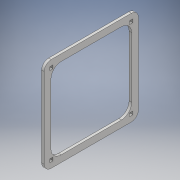
# Autodesk Inventor part: FrontPanelSquishything
Saved by Autodesk Inventor 2017 (Build 210142000, 142)
## iProperties
Created: 2019-07-06
Part Number: FrontPanelSquishything
Material: Generic
Document SubType Name: Modeling
Designer: DDeGo
Density: 1 g/cm^3
Appearance: Default
Author: DDeGo
Autodesk Inventor part; units mm, degrees
ref_plane "YZ Plane" through (0, 0, 0) normal (1, 0, 0) x (0, 1, 0)
ref_plane "XZ Plane" through (0, 0, 0) normal (0, 1, 0) x (-1, 0, 0)
ref_plane "XY Plane" through (0, 0, 0) normal (0, 0, 1) x (1, 0, 0)
sketch "Sketch1" plane through (0, 0, 0) normal (1, 0, 0) x (0, 1, 0)
  line L0 (0, 13.5) -> (156.2, 13.5)
  line L1 (169.7, 0) -> (169.7, -156.2)
  line L2 (156.2, -169.7) -> (0, -169.7)
  line L3 (-13.5, -156.2) -> (-13.5, 0)
  arc A0 (169.7, 0) -> (156.2, 13.5) centre (156.2, 0) ccw
  arc A1 (156.2, -169.7) -> (169.7, -156.2) centre (156.2, -156.2) ccw
  arc A2 (-13.5, -156.2) -> (0, -169.7) centre (0, -156.2) ccw
  arc A3 (0, 13.5) -> (-13.5, 0) centre (0, 0) ccw
  line L4 (19.5, 0.5) -> (136.7, 0.5)
  line L5 (156.7, -19.5) -> (156.7, -136.7)
  line L6 (136.7, -156.7) -> (19.5, -156.7)
  line L7 (-0.5, -136.7) -> (-0.5, -19.5)
  arc A4 (19.5, 0.5) -> (-0.5, -19.5) centre (19.5, -19.5) ccw
  arc A5 (-0.5, -136.7) -> (19.5, -156.7) centre (19.5, -136.7) ccw
  arc A6 (136.7, -156.7) -> (156.7, -136.7) centre (136.7, -136.7) ccw
  arc A7 (156.7, -19.5) -> (136.7, 0.5) centre (136.7, -19.5) ccw
  dimension "d0" = 13.5
  dimension "d1" = 183.2
  dimension "d2" = 183.2
  dimension "d15" = 13
  dimension "d16" = 13
  dimension "d17" = 13
  dimension "d18" = 13
  dimension "d19" = 20
  constraints: 16 end point, 16 point on circle, 16 tangent, 8 centre point, 6 equal radius, 4 parallel, 2 horizontal, 2 perpendicular, 1 other
  measures "d0" radius of A0
  measures "d1" distance between parallel lines of L2 L0
  measures "d2" distance between parallel lines of L1 L3
  measures "d15" distance between parallel lines of L3 L7
  measures "d16" distance between parallel lines of L0 L4
  measures "d17" distance between parallel lines of L1 L5
  measures "d18" distance between parallel lines of L2 L6
  measures "d19" radius of A4
extrude "Extrusion1" add sketch "Sketch1" along normal blind 5
sketch "Sketch2" plane through (0, 0, 0) normal (-1, 0, 0) x (0, 0, 1)
  line L0 (-0.5, 155.7) -> (-155.7, 155.7) construction
  line L1 (-155.7, 155.7) -> (-155.7, 0.5) construction
  line L2 (-155.7, 0.5) -> (-0.5, 0.5) construction
  line L3 (-0.5, 0.5) -> (-0.5, 155.7) construction
  line L4 (2.625, 152.575) -> (-3.625, 152.575)
  line L5 (-3.625, 152.575) -> (-3.625, 158.825)
  line L6 (-3.625, 158.825) -> (2.625, 158.825)
  line L7 (2.625, 158.825) -> (2.625, 152.575)
  line L8 (2.625, 152.575) -> (-3.625, 158.825) construction
  line L9 (-3.625, 152.575) -> (2.625, 158.825) construction
  line L10 (-3.625, 3.625) -> (2.625, 3.625)
  line L11 (2.625, 3.625) -> (2.625, -2.625)
  line L12 (2.625, -2.625) -> (-3.625, -2.625)
  line L13 (-3.625, -2.625) -> (-3.625, 3.625)
  line L14 (-3.625, 3.625) -> (2.625, -2.625) construction
  line L15 (2.625, 3.625) -> (-3.625, -2.625) construction
  line L16 (-158.825, 3.625) -> (-152.575, 3.625)
  line L17 (-152.575, 3.625) -> (-152.575, -2.625)
  line L18 (-152.575, -2.625) -> (-158.825, -2.625)
  line L19 (-158.825, -2.625) -> (-158.825, 3.625)
  line L20 (-158.825, 3.625) -> (-152.575, -2.625) construction
  line L21 (-152.575, 3.625) -> (-158.825, -2.625) construction
  line L22 (-152.575, 152.575) -> (-158.825, 152.575)
  line L23 (-158.825, 152.575) -> (-158.825, 158.825)
  line L24 (-158.825, 158.825) -> (-152.575, 158.825)
  line L25 (-152.575, 158.825) -> (-152.575, 152.575)
  line L26 (-152.575, 152.575) -> (-158.825, 158.825) construction
  line L27 (-158.825, 152.575) -> (-152.575, 158.825) construction
  line L28 (-156.2, -13.5) -> (0, -13.5) projected
  line L29 (13.5, 0) -> (13.5, 156.2) projected
  line L30 (0, 169.7) -> (-156.2, 169.7) projected
  line L31 (-169.7, 156.2) -> (-169.7, 0) projected
  point P0 (0, 0)
  dimension "d20" = 6.25
  dimension "d21" = 6.25
  dimension "d22" = 14
  dimension "d23" = 14
  dimension "d24" = 14
  dimension "d25" = 14
  constraints: 56 end point, 10 parallel, 8 midpoint, 6 equal length, 5 horizontal, 5 perpendicular
  measures "d20" distance of L5.end L6.end
  measures "d21" distance of L6.end L4.start
  measures "d22" distance between parallel lines of L28 L2
  measures "d23" distance between parallel lines of L29 L3
  measures "d24" distance between parallel lines of L30 L0
  measures "d25" distance between parallel lines of L31 L1
extrude "Extrusion2" cut sketch "Sketch2" against normal blind 10
equation "\"d1\" = d2"
equation "\"d16\" = d15"
equation "\"d17\" = d15"
equation "\"d18\" = d15"
equation "\"d22\" = d23"
equation "\"d24\" = d23"
equation "\"d25\" = d23"
body "Solid1"
